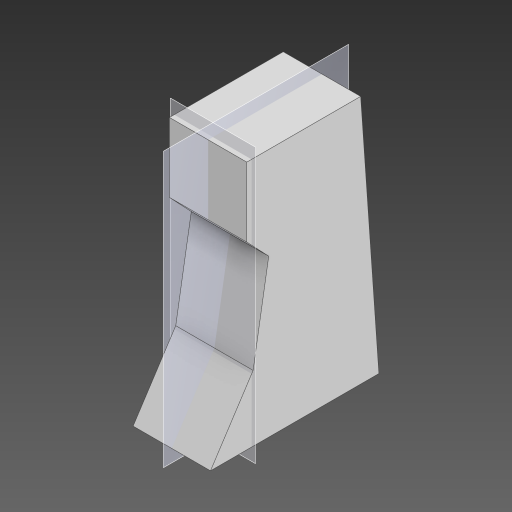
# Autodesk Inventor part: BaseBoundingBox
Saved by Autodesk Inventor 2023 (Build 270158000, 158)
## iProperties
Created: 2023-03-19
Part Number: BaseBoundingBox
Material: Generic
Document SubType Name: Modeling
Designer: Val
Density: 1 g/cm^3
Appearance: Default
Author: Val
Autodesk Inventor part; units mm, degrees
ref_plane "XZ Plane" through (0, 0, 0) normal (0, 1, 0) x (-1, 0, 0)
sketch "Sketch1" plane through (0, 0, 0) normal (1, 0, 0) x (0, 1, 0)
  line L0 (-136.2516, 26.0681) -> (-94.6911, -0.9217)
  line L1 (-94.6911, -0.9217) -> (-36.9927, -10.7705)
  line L2 (-36.9927, -10.7705) -> (-22.35, 3.08)
  line L3 (-22.35, 3.08) -> (21.5, 3.08)
  line L4 (21.5, 3.08) -> (21.5, -69)
  line L5 (21.5, -69) -> (-136.2516, -80.5428)
  line L6 (-136.2516, -80.5428) -> (-136.2516, 26.0681)
  line L7 (-20.328, 3.08) -> (15.75, 3.08)
  line L8 (21.5, 2) -> (21.5, -10)
  line L9 (-36.9927, -10.7705) -> (-23.8189, 1.6905)
  line L10 (-136.2516, -70.0311) -> (-136.2516, 7.0311)
  line L11 (-120.3625, 15.7495) -> (-94.6911, -0.9217)
  point P0 (0, 0)
  point P1 (-136.2516, 7.0311)
  dimension "d0" = 46.592
  dimension "d1" = 94.185
  dimension "d2" = 99.687
  dimension "d3" = 57
  dimension "d4" = 157.7516
  dimension "d5" = 21.5
  dimension "d6" = 3.08
  dimension "d7" = 17.5961
  dimension "d8" = 70.385
  dimension "d9" = 16.8414
  dimension "d10" = 52.3454
  dimension "d11" = 1.08
  dimension "d12" = 13.08
  dimension "d13" = 5.75
  dimension "d14" = 41.828
  dimension "d15" = 45.3189
  dimension "d16" = 141.8624
  dimension "d17" = 3.9511
  dimension "d18" = 73.1111
  constraints: 24 end point, 5 collinear, 1 coincident, 1 horizontal, 1 parallel, 1 perpendicular
  measures "d0" angle of L4 L9
  measures "d1" angle of L4 L5
  measures "d2" angle of L4 L1
  measures "d3" angle of L4 L0
  measures "d4" distance between parallel lines of L4 L6
  measures "d5" distance from line of point (0, 0) L4
  measures "d6" distance from line of point (0, 0) L3
  measures "d7" distance from line of point (0, 0) L9
  measures "d8" distance from line of point (0, 0) L5
  measures "d9" distance from line of point (0, 0) L1
  measures "d10" distance from line of point (0, 0) L0
  measures "d11" distance from line of L8.start L3
  measures "d12" distance from line of L8.end L3
  measures "d13" distance from line of L7.end L4
  measures "d14" distance from line of L7.start L4
  measures "d15" distance from line of L9.end L4
  measures "d16" distance from line of L11.start L4
  measures "d17" distance from line of L10.end L3
  measures "d18" distance from line of L10.start L3
extrude "Extrusion1" add sketch "Sketch1" along normal mid plane 48.9966
body "Solid1"
